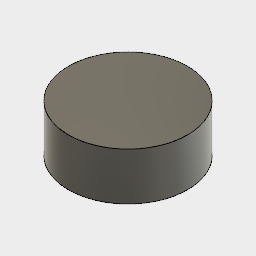
cylinder to fix platform (Autodesk Fusion 360 design; units mm, degrees)
Autodesk Fusion 360 part; units mm, degrees
sketch "Sketch1" plane through (0, 0, 0) normal (0, 0, 1) x (1, 0, 0)
  line L0 (0.0004, 4.4623) -> (7.1161, 4.4623)
  line L1 (7.1161, 1.4623) -> (7.1161, 4.4623)
  line L2 (7.1161, 1.4623) -> (12.5004, 1.4623)
  line L3 (12.5004, 1.4623) -> (12.5004, 11.4623)
  line L4 (12.5004, 11.4623) -> (0.0004, 11.4623)
  line L5 (0.0004, 11.4623) -> (0.0004, 4.4623)
  dimension "d4" = 3
  dimension "d5" = 10
  dimension "d6" = 12.5
  measures "d4" distance of L0.end L1.start
  measures "d5" distance of L2.end L3.end
  measures "d6" distance of L3.end L4.end
revolve "Revolve1" add sketch "Sketch1" angle 360 about axis through (0, 1.75, 0) along (0, 1, 0)
